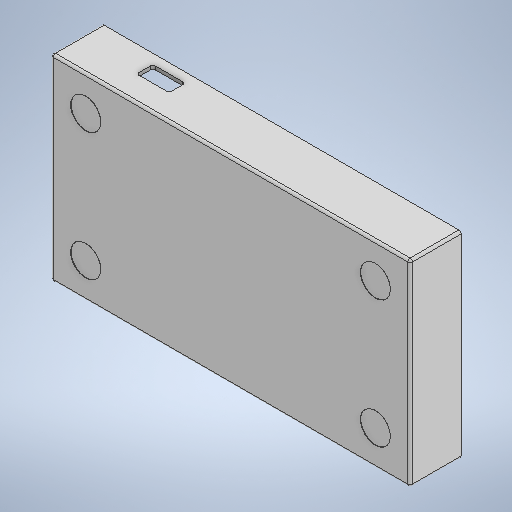
# Autodesk Inventor part: Datapad_Case
Saved by Autodesk Inventor 2025 (Build 290162000, 162)
## iProperties
Created: 2026-06-22
Part Number: Datapad_Case
Material: Generisch
Document SubType Name: Modeling
Designer: plauffs
Density: 1 g/cm^3
Appearance: Vorgabe
Author: plauffs
Autodesk Inventor part; units mm, degrees
ref_plane "YZ Plane" through (0, 0, 0) normal (1, 0, 0) x (0, 1, 0)
ref_plane "XZ Plane" through (0, 0, 0) normal (0, 1, 0) x (-1, 0, 0)
ref_plane "XY Plane" through (0, 0, 0) normal (0, 0, 1) x (1, 0, 0)
sketch "Skizze1" plane through (0, 0, 0) normal (0, 1, 0) x (-1, 0, 0)
  line L0 (0, 0) -> (155, 0)
  line L1 (155, 0) -> (155, -85)
  line L2 (155, -85) -> (0, -85)
  line L3 (0, -85) -> (0, 0)
  dimension "d0" = 155
  dimension "d1" = 85
  constraints: 8 end point, 2 parallel, 1 horizontal, 1 perpendicular
  measures "d0" distance of L1.end L2.end
  measures "d1" distance of L0.end L1.end
extrude "Extrusion1" add sketch "Skizze1" along normal blind 22
sketch "Skizze2" plane through (0, 22, 0) normal (0, 1, 0) x (1, 0, 0)
  line L0 (-1.5, 1.5) -> (-153.5, 1.5)
  line L1 (-153.5, 1.5) -> (-153.5, 83.5)
  line L2 (-153.5, 83.5) -> (-1.5, 83.5)
  line L3 (-1.5, 83.5) -> (-1.5, 1.5)
  line L4 (-155, 0) -> (0, 0) projected
  line L5 (0, 85) -> (-155, 85) projected
  line L6 (0, 0) -> (0, 85) projected
  line L7 (-155, 85) -> (-155, 0) projected
  dimension "d4" = 1.5
  dimension "d5" = 1.5
  dimension "d6" = 1.5
  dimension "d7" = 1.5
  constraints: 8 end point, 2 parallel, 1 horizontal, 1 perpendicular
  measures "d4" distance between parallel lines of L4 L0
  measures "d5" distance between parallel lines of L5 L2
  measures "d6" distance between parallel lines of L6 L3
  measures "d7" distance between parallel lines of L7 L1
extrude "Extrusion2" cut sketch "Skizze2" against normal blind 20.5 contours L0 L1 L2 L3
sketch "Skizze3" plane through (-155, 0, 0) normal (0, 0, 1) x (1, 0, 0)
  line L0 (27.2, 17.8) -> (39.2, 17.8)
  line L1 (40.2, 16.8) -> (40.2, 11.8)
  line L2 (39.2, 10.8) -> (27.2, 10.8)
  line L3 (26.2, 11.8) -> (26.2, 16.8)
  arc A0 (26.2, 11.8) -> (27.2, 10.8) centre (27.2, 11.8) ccw
  arc A1 (27.2, 17.8) -> (26.2, 16.8) centre (27.2, 16.8) ccw
  arc A2 (40.2, 16.8) -> (39.2, 17.8) centre (39.2, 16.8) ccw
  arc A3 (39.2, 10.8) -> (40.2, 11.8) centre (39.2, 11.8) ccw
  line L4 (153.5, 1.5) -> (1.5, 1.5) projected
  line L5 (1.5, 22) -> (1.5, 1.5) projected
  point P0 (155, 0)
  dimension "d10" = 1
  dimension "d71" = 14
  dimension "d72" = 7
  dimension "d73" = 9.3
  dimension "d74" = 24.7
  constraints: 8 end point, 8 point on circle, 8 tangent, 4 centre point, 3 equal radius, 2 parallel, 1 horizontal, 1 perpendicular
  measures "d10" radius of A0
  measures "d71" distance between parallel lines of L1 L3
  measures "d72" distance between parallel lines of L2 L0
  measures "d73" distance between parallel lines of L4 L2
  measures "d74" distance between parallel lines of L5 L3
extrude "Extrusion3" cut sketch "Skizze3" against normal blind 3
sketch "Skizze4" plane through (0, 1.5, 0) normal (0, 1, 0) x (1, 0, 0)
  circle A0 centre (-80.95, 23.5) radius 2.75
  circle A1 centre (-80.95, 61.5) radius 2.75
  circle A2 centre (-23.95, 23.5) radius 2.75
  circle A3 centre (-23.95, 61.5) radius 2.75
  circle A4 centre (-80.95, 23.5) radius 1.2
  circle A5 centre (-80.95, 61.5) radius 1.2
  circle A6 centre (-23.95, 23.5) radius 1.2
  circle A7 centre (-23.95, 61.5) radius 1.2
  line L0 (-1.5, 83.5) -> (-1.5, 1.5) projected
  line L1 (-1.5, 1.5) -> (-153.5, 1.5) projected
  line L2 (-153.5, 83.5) -> (-1.5, 83.5) projected
  point P0 (0, 0)
  dimension "d13" = 5.5
  dimension "d14" = 5.5
  dimension "d15" = 5.5
  dimension "d16" = 5.5
  dimension "d17" = 38
  dimension "d18" = 38
  dimension "d19" = 57
  dimension "d40" = 2.4
  dimension "d41" = 2.4
  dimension "d42" = 2.4
  dimension "d43" = 2.4
  dimension "d44" = 22.45
  dimension "d45" = 22
  dimension "d47" = 22
  dimension "d51" = 22.45
  dimension "d53" = 57
  dimension "d54" = 22
  dimension "d55" = 22
  constraints: 8 centre point, 4 coincident
  measures "d13" diameter of A0
  measures "d14" diameter of A1
  measures "d15" diameter of A2
  measures "d16" diameter of A3
  measures "d17" distance of A1.centre A0.centre
  measures "d18" distance of A3.centre A2.centre
  measures "d19" distance of A2.centre A0.centre
  measures "d40" diameter of A4
  measures "d41" diameter of A5
  measures "d42" diameter of A6
  measures "d43" diameter of A7
  measures "d44" distance from line of L0 A2.centre
  measures "d45" distance from line of L1 A0.centre
  measures "d47" distance from line of L1 A2.centre
  measures "d51" distance from line of L0 A3.centre
  measures "d53" distance of A3.centre A1.centre
  measures "d54" distance from line of L2 A3.centre
  measures "d55" distance from line of L2 A5.centre
extrude "Extrusion4" add sketch "Skizze4" along normal blind 5.5
sketch "Skizze5" plane through (-155, 0, -85) normal (-1, 0, 0) x (0, 0, 1)
  line L0 (15.5, 8.6) -> (24.5, 8.6)
  line L1 (24.5, 8.6) -> (24.5, 13.6)
  line L2 (24.5, 13.6) -> (15.5, 13.6)
  line L3 (15.5, 13.6) -> (15.5, 8.6)
  line L4 (1.5, 22) -> (1.5, 1.5) projected
  line L5 (83.5, 1.5) -> (1.5, 1.5) projected
  point P0 (85, 0)
  dimension "d59" = 14
  dimension "d60" = 9
  dimension "d61" = 5
  dimension "d62" = 7.1
  constraints: 8 end point, 2 parallel, 1 horizontal, 1 perpendicular
  measures "d59" distance between parallel lines of L4 L3
  measures "d60" distance of L1.end L2.end
  measures "d61" distance of L0.end L1.end
  measures "d62" distance between parallel lines of L5 L0
extrude "Extrusion5" cut sketch "Skizze5" against normal blind 3
fillet "Rundung1" radius 1 4 edges at (0, 11, 0) (0, 11, -85) (-155, 11, 0) (-155, 11, -85)
fillet "Rundung2" radius 1 8 edges at (-0.2929, 0, -0.2929) (0, 0, -42.5) (-0.2929, 0, -84.7071) (-77.5, 0, -85) (-154.7071, 0, -84.7071) (-155, 0, -42.5) (-154.7071, 0, -0.2929) (-77.5, 0, 0)
sketch "Skizze6" plane through (0, 0, 0) normal (0, -1, 0) x (1, 0, 0)
  circle A0 centre (-140, -70) radius 6.5
  circle A1 centre (-140, -15) radius 6.5
  circle A2 centre (-15, -70) radius 6.5
  circle A3 centre (-15, -15) radius 6.5
  line L0 (-1, 0) -> (-154, 0) projected
  line L1 (-154, -85) -> (-1, -85) projected
  line L2 (-155, -1) -> (-155, -84) projected
  line L3 (0, -84) -> (0, -1) projected
  point P0 (0, 0)
  dimension "d26" = 13
  dimension "d27" = 13
  dimension "d28" = 13
  dimension "d29" = 13
  dimension "d63" = 15
  dimension "d64" = 15
  dimension "d65" = 15
  dimension "d66" = 15
  dimension "d67" = 15
  dimension "d68" = 15
  dimension "d69" = 15
  dimension "d70" = 15
  constraints: 4 centre point
  measures "d26" diameter of A0
  measures "d27" diameter of A1
  measures "d28" diameter of A2
  measures "d29" diameter of A3
  measures "d63" distance from line of L0 A1.centre
  measures "d64" distance from line of L1 A0.centre
  measures "d65" distance from line of L0 A3.centre
  measures "d66" distance from line of L1 A2.centre
  measures "d67" distance from line of L2 A0.centre
  measures "d68" distance from line of L2 A1.centre
  measures "d69" distance from line of L3 A2.centre
  measures "d70" distance from line of L3 A3.centre
extrude "Extrusion6" cut sketch "Skizze6" against normal blind 0.2
sketch "Skizze7" plane through (-1, 22, -85) normal (0, 0, -1) x (-1, 0, 0)
  circle A0 centre (128.2, -10) radius 1.5
  circle A1 centre (117.6, -10) radius 1.5
  line L0 (152.5, -20.5) -> (0.5, -20.5) projected
  line L1 (152.5, 0) -> (152.5, -20.5) projected
  point P0 (-1, -22)
  dimension "d35" = 3
  dimension "d36" = 3
  dimension "d37" = 10.6
  dimension "d56" = 10.5
  dimension "d57" = 10.5
  dimension "d58" = 24.3
  constraints: 2 centre point
  measures "d35" diameter of A1
  measures "d36" diameter of A0
  measures "d37" distance of A0.centre A1.centre
  measures "d56" distance from line of L0 A1.centre
  measures "d57" distance from line of L0 A0.centre
  measures "d58" distance from line of L1 A0.centre
extrude "Extrusion7" cut sketch "Skizze7" against normal blind 3
